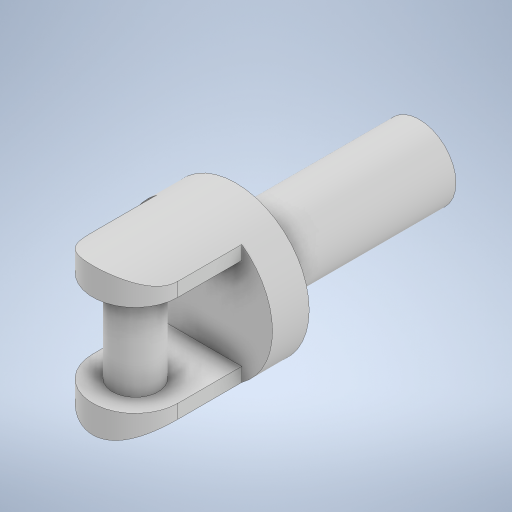
# Autodesk Inventor part: u_joint
Saved by Autodesk Inventor 2023 (Build 270158000, 158)
## iProperties
Created: 2023-09-13
Part Number: u_joint
Material: Generic
Document SubType Name: Modeling
Designer: Peter
Density: 1 g/cm^3
Appearance: Default
Author: Peter
Autodesk Inventor part; units mm, degrees
ref_plane "YZ Plane" through (0, 0, 0) normal (1, 0, 0) x (0, 1, 0)
ref_plane "XZ Plane" through (0, 0, 0) normal (0, 1, 0) x (-1, 0, 0)
ref_plane "XY Plane" through (0, 0, 0) normal (0, 0, 1) x (1, 0, 0)
sketch "Sketch1" plane through (0, 0, 0) normal (0, 0, 1) x (1, 0, 0)
  circle A0 centre (0, 0) radius 25.4
  dimension "d0" = 50.8
  constraints: 1 centre point, 1 coincident
  measures "d0" diameter of A0
extrude "Extrusion1" add sketch "Sketch1" along normal blind 25.4 and the other way blind 101.6
sketch "Sketch2" plane through (0, 0, 0) normal (0, 1, 0) x (-1, 0, 0)
  line L0 (0, -25.4) -> (0, 152.4) construction
  line L1 (25.4, 25.4) -> (-25.4, 25.4) construction
  line L2 (0, 25.4) -> (-50.8, 25.4)
  line L3 (-50.8, 25.4) -> (-50.8, 127)
  line L4 (-50.8, 127) -> (0, 127)
  line L5 (0, 127) -> (0, 25.4)
  point P0 (0, 0)
  dimension "d8" = 50.8
  dimension "d9" = 101.6
  constraints: 8 end point, 2 parallel, 1 horizontal, 1 midpoint, 1 perpendicular
  measures "d8" distance of L3.end L4.end
  measures "d9" distance of L2.end L3.end
revolve "Revolution1" add sketch "Sketch2" angle 360 about axis through (0, 0, -10) along (0, 0, 1)
sketch "Sketch3" plane through (0, 0, 0) normal (1, 0, 0) x (0, 1, 0)
  line L0 (50.8, 127) -> (-50.8, 127) construction
  line L1 (31.75, 127) -> (-31.75, 127)
  line L2 (-31.75, 127) -> (-31.75, 50.8)
  line L3 (-31.75, 50.8) -> (31.75, 50.8)
  line L4 (31.75, 50.8) -> (31.75, 127)
  line L5 (0, -25.4) -> (0, 152.4) construction
  point P0 (0, 0)
  point P1 (0, 50.8)
  dimension "d11" = 0
  dimension "d12" = 76.2
  dimension "d13" = 63.5
  constraints: 8 end point, 2 parallel, 1 horizontal, 1 midpoint, 1 perpendicular, 1 point on line
  measures "d11" distance from line of point (0, 50.8) L5
  measures "d12" distance of L1.end L2.end
  measures "d13" distance of L2.end L3.end
extrude "Extrusion2" cut sketch "Sketch3" along normal mid plane 254
sketch "Sketch4" plane through (0, 0, 0) normal (0, 1, 0) x (-1, 0, 0)
  line L0 (-39.6557, 127) -> (39.6557, 127) construction
  line L1 (39.6557, 127) -> (39.6557, 50.8) construction
  line L2 (-39.6557, 50.8) -> (-39.6557, 127) construction
  line L3 (-29.4957, 50.8) -> (-29.4957, 94.9643)
  line L4 (39.6557, 50.8) -> (-39.6557, 50.8) construction
  line L5 (29.4957, 94.9643) -> (29.4957, 50.8)
  arc A0 (29.4957, 94.9643) -> (-29.4957, 94.9643) centre (0, 94.9643) ccw
  line L6 (-29.4957, 50.8) -> (-112.68, 50.8)
  line L7 (-112.68, 50.8) -> (-112.68, 137.8838)
  line L8 (-112.68, 137.8838) -> (83.0957, 137.8838)
  line L9 (83.0957, 137.8838) -> (83.0957, 50.8)
  line L10 (83.0957, 50.8) -> (29.4957, 50.8)
  line L11 (39.6557, 127) -> (-39.6557, 127) construction
  point P0 (0, 0)
  point P1 (0, 124.46)
  point P2 (0, 127)
  point P3 (0, 127)
  dimension "d16" = 10.16
  dimension "d17" = 10.16
  dimension "d24" = 2.54
  constraints: 14 end point, 5 perpendicular, 3 point on circle, 2 midpoint, 2 point on line, 2 tangent, 1 centre point, 1 horizontal, 1 vertical
  measures "d16" distance between parallel lines of L2 L3
  measures "d17" distance between parallel lines of L1 L5
  measures "d24" distance of point (0, 127) point (0, 124.46)
extrude "Extrusion3" cut sketch "Sketch4" along normal mid plane 254
sketch "Sketch5" plane through (0, 31.75, 94.9643) normal (0, -1, 0) x (1, 0, 0)
  circle A0 centre (0, 0) radius 15.875
  line L0 (29.4957, 0) -> (29.4957, -44.1643) construction
  line L1 (-29.4957, 0) -> (29.4957, 0) construction
  point P0 (0, -94.9643)
  dimension "d21" = 31.75
  constraints: 2 end point, 1 centre point, 1 coincident, 1 horizontal, 1 midpoint
  measures "d21" diameter of A0
extrude "Extrusion4" add sketch "Sketch5" along normal up to next
body "Solid1"
